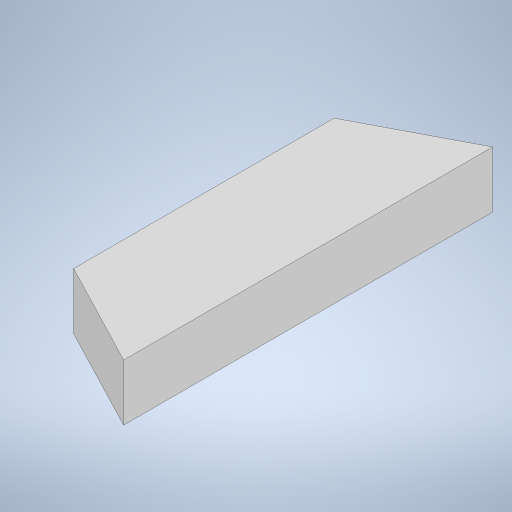
# Autodesk Inventor part: ButtonPanel
Saved by Autodesk Inventor 2023 (Build 270158000, 158)
## iProperties
Created: 2024-03-26
Part Number: ButtonPanel
Material: Generic
Document SubType Name: Modeling
Designer: noname
Density: 1 g/cm^3
Appearance: Default
Author: noname
Autodesk Inventor part; units mm, degrees
ref_plane "YZ Plane" through (0, 0, 0) normal (1, 0, 0) x (0, 1, 0)
ref_plane "XZ Plane" through (0, 0, 0) normal (0, 1, 0) x (-1, 0, 0)
ref_plane "XY Plane" through (0, 0, 0) normal (0, 0, 1) x (1, 0, 0)
sketch "Sketch1" plane through (0, 0, 0) normal (0, 1, 0) x (-1, 0, 0)
  line L0 (0, 0) -> (0, -85)
  line L1 (0, -85) -> (24, -72.5)
  line L2 (24, -72.5) -> (24, -12.5)
  line L3 (24, -12.5) -> (0, 0)
  dimension "d1" = 24
  dimension "d2" = 85
  dimension "d3" = 60
  constraints: 8 end point, 1 equal length, 1 parallel, 1 vertical
  measures "d1" distance between parallel lines of L0 L2
  measures "d2" distance of L0.start L0.end
  measures "d3" distance of L1.end L2.end
extrude "Extrusion1" add sketch "Sketch1" along normal blind 13
body "Solid1"
